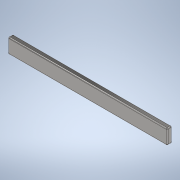
# Autodesk Inventor part: Chassis base shaft
Saved by Autodesk Inventor 2020 (Build 240168000, 168)
## iProperties
Created: 2022-07-02
Part Number: Chassis base shaft
Material: Generic
Document SubType Name: Modeling
Designer: karimi2
Density: 1 g/cm^3
Appearance: Steel - Polished
Author: karimi2
Autodesk Inventor part; units mm, degrees
ref_plane "YZ Plane" through (0, 0, 0) normal (1, 0, 0) x (0, 1, 0)
ref_plane "XZ Plane" through (0, 0, 0) normal (0, 1, 0) x (-1, 0, 0)
ref_plane "XY Plane" through (0, 0, 0) normal (0, 0, 1) x (1, 0, 0)
sketch "Sketch1" plane through (0, 0, 0) normal (0, 0, 1) x (1, 0, 0)
  line L0 (0, 0) -> (320, 0)
  line L1 (320, 0) -> (320, 30)
  line L2 (320, 30) -> (0, 30)
  line L3 (0, 30) -> (0, 0)
  dimension "d0" = 320
  dimension "d1" = 30
  constraints: 8 end point, 2 parallel, 1 horizontal, 1 perpendicular
  measures "d0" distance of L1.end L2.end
  measures "d1" distance of L0.end L1.end
extrude "Extrusion1" add sketch "Sketch1" along normal mid plane 10
fillet "Fillet1" radius 2 12 edges at (160, 30, 5) (160, 30, -5) (160, 0, 5) (320, 15, 5) (320, 15, -5) (320, 30, 0) (320, 0, 0) (160, 0, -5) (0, 30, 0) (0, 15, 5) (0, 15, -5) (0, 0, 0)
body "Solid1"
